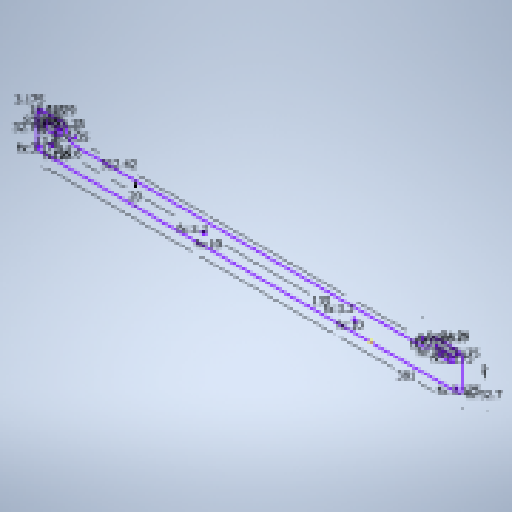
# Autodesk Inventor part: Middle Slide
Saved by Autodesk Inventor 2023 (Build 270158000, 158)
## iProperties
Created: 2022-09-10
Part Number: Middle Slide
Material: Generic
Document SubType Name: Modeling
Designer: deli
Density: 1 g/cm^3
Appearance: Default
Author: deli
Autodesk Inventor part; units mm, degrees
ref_plane "YZ Plane" through (0, 0, 0) normal (1, 0, 0) x (0, 1, 0)
ref_plane "XZ Plane" through (0, 0, 0) normal (0, 1, 0) x (-1, 0, 0)
ref_plane "XY Plane" through (0, 0, 0) normal (0, 0, 1) x (1, 0, 0)
sketch "Sketch1" plane through (0, 0, 0) normal (0, 0, 1) x (1, 0, 0)
  arc A0 (81, 29.525) -> (77.825, 32.7) centre (77.825, 29.525) ccw
  line L0 (77.825, 32.7) -> (59.41, 32.7)
  arc A1 (59.41, 32.7) -> (53.06, 26.35) centre (59.41, 26.35) ccw
  arc A2 (46.71, 20) -> (53.06, 26.35) centre (46.71, 26.35) ccw
  line L1 (46.71, 20) -> (-265.71, 20)
  arc A3 (-272.06, 26.35) -> (-265.71, 20) centre (-265.71, 26.35) ccw
  arc A4 (-272.06, 26.35) -> (-278.41, 32.7) centre (-278.41, 26.35) ccw
  line L2 (-278.41, 32.7) -> (-296.825, 32.7)
  arc A5 (-296.825, 32.7) -> (-300, 29.525) centre (-296.825, 29.525) ccw
  line L3 (-300, 29.525) -> (-300, 3.175)
  arc A6 (-300, 3.175) -> (-296.825, 0) centre (-296.825, 3.175) ccw
  line L4 (-296.825, 0) -> (77.825, 0)
  arc A7 (77.825, 0) -> (81, 3.175) centre (77.825, 3.175) ccw
  line L5 (81, 3.175) -> (81, 29.525)
  arc A8 (62.585, 26.35) -> (62.585, 20) centre (62.585, 23.175) ccw
  line L6 (62.585, 26.35) -> (71.475, 26.35)
  arc A9 (71.475, 20) -> (71.475, 26.35) centre (71.475, 23.175) ccw
  line L7 (71.475, 20) -> (62.585, 20)
  line L8 (-290.475, 26.35) -> (-281.585, 26.35)
  arc A10 (-281.585, 20) -> (-281.585, 26.35) centre (-281.585, 23.175) ccw
  line L9 (-281.585, 20) -> (-290.475, 20)
  arc A11 (-290.475, 26.35) -> (-290.475, 20) centre (-290.475, 23.175) ccw
  circle A12 centre (-151.6, 10) radius 1.6
  circle A13 centre (-286.6, 10) radius 1.6
  circle A14 centre (-16.6, 10) radius 1.6
  point P0 (0, 0)
  point P1 (-272.06, 26.35)
  point P2 (-300, 3.175)
  point P3 (-296.825, 0)
  point P4 (77.825, 0)
  point P5 (62.585, 26.35)
  dimension "d0" = 3.175
  dimension "d1" = 6.35
  dimension "d2" = 3.175
  dimension "d3" = 3.175
  dimension "d4" = 32.7
  dimension "d5" = 34.29
  dimension "d6" = 6.35
  dimension "d7" = 381
  dimension "d8" = 312.42
  dimension "d9" = 34.29
  dimension "d10" = 32.7
  dimension "d11" = 3.175
  dimension "d12" = 3.175
  dimension "d13" = 3.2
  dimension "d14" = 3.2
  dimension "d15" = 3.2
  dimension "d16" = 20
  dimension "d17" = 6.35
  dimension "d18" = 13.4
  dimension "d19" = 10
  dimension "d20" = 10
  dimension "d21" = 10
  dimension "d22" = 6.35
  dimension "d23" = 9.525
  dimension "d24" = 8.89
  dimension "d25" = 3.175
  dimension "d26" = 3.175
  dimension "d27" = 3.175
  dimension "d28" = 6.35
  dimension "d29" = 6.35
  dimension "d30" = 18.415
  dimension "d31" = 18.415
  dimension "d32" = 135
  dimension "d33" = 135
  constraints: 24 point on circle, 20 end point, 15 centre point, 2 tangent, 1 perpendicular
  measures "d0" radius of A5
  measures "d1" radius of A4
  measures "d2" radius of A11
  measures "d3" radius of A10
  measures "d4" distance between parallel lines of L4 L2
  measures "d5" distance from line of L1.end L3
  measures "d6" radius of A3
  measures "d7" distance between parallel lines of L5 L3
  measures "d8" distance of L1.start L1.end
  measures "d9" distance from line of L5 A2.start
  measures "d10" distance between parallel lines of L4 L0
  measures "d11" radius of A8
  measures "d12" radius of A9
  measures "d13" diameter of A13
  measures "d14" diameter of A12
  measures "d15" diameter of A14
  measures "d16" distance between parallel lines of L4 L1
  measures "d17" distance between parallel lines of L8 L9
  measures "d18" distance from line of A13.centre L3
  measures "d19" distance from line of L4 A13.centre
  measures "d20" distance from line of L4 A12.centre
  measures "d21" distance from line of L4 A14.centre
  measures "d22" distance between parallel lines of L2 L8
  measures "d23" distance from line of L3 A11.centre
  measures "d24" distance of L8.start L8.end
  measures "d25" radius of A6
  measures "d26" radius of A7
  measures "d27" radius of A0
  measures "d28" radius of A1
  measures "d29" radius of A2
  measures "d30" distance of L2.start L2.end
  measures "d31" distance of L0.start L0.end
  measures "d32" distance of A13.centre A12.centre
  measures "d33" distance of A14.centre A12.centre
extrude "Extrusion1" add sketch "Sketch1" along normal blind 6.35
sketch "Sketch2" plane through (-296.825, 32.7, 0) normal (0, 1, 0) x (1, 0, 0)
  line L0 (18.415, 0) -> (0, 0) projected
  line L1 (0, 0) -> (0, -6.35) projected
  line L2 (18.415, -6.35) -> (0, -6.35) projected
  line L3 (18.415, 0) -> (18.415, -6.35) projected
  line L4 (374.65, 0) -> (356.235, 0) projected
  line L5 (356.235, 0) -> (356.235, -6.35) projected
  line L6 (374.65, -6.35) -> (356.235, -6.35) projected
  line L7 (374.65, 0) -> (374.65, -6.35) projected
  circle A0 centre (365.4425, -3.175) radius 1.5
  circle A1 centre (9.2075, -3.175) radius 1.5
  point P0 (296.825, 0)
  dimension "d36" = 3
  dimension "d37" = 3
  dimension "d38" = 3.175
  dimension "d39" = 6.35
  dimension "d40" = 18.415
  dimension "d41" = 9.2075
  dimension "d42" = 3.175
  dimension "d43" = 9.2075
  constraints: 2 centre point
  measures "d36" diameter of A0
  measures "d37" diameter of A1
  measures "d38" distance from line of L0 A1.centre
  measures "d39" distance of L0.end L1.end
  measures "d40" distance of L0.start L0.end
  measures "d41" distance from line of L1 A1.centre
  measures "d42" distance from line of L4 A0.centre
  measures "d43" distance from line of L5 A0.centre
extrude "Extrusion2" cut sketch "Sketch2" against normal blind 20 contours A0 | A1
equation "\"d3\" = d2"
equation "\"d6\" = d1"
equation "\"d9\" = d5"
equation "\"d10\" = d4"
equation "\"d11\" = d2"
equation "\"d12\" = d2"
equation "\"d14\" = d13"
equation "\"d15\" = d13"
equation "\"d19\" = 0.5 * d16"
equation "\"d20\" = d19"
equation "\"d21\" = d19"
equation "\"d25\" = d0"
equation "\"d26\" = d0"
equation "\"d27\" = d0"
equation "\"d28\" = d1"
equation "\"d29\" = d1"
equation "\"d31\" = d30"
equation "\"d33\" = d32"
equation "\"d38\" = 0.5 * d39"
equation "\"d41\" = 0.5 * d40"
equation "\"d42\" = d38"
equation "\"d43\" = d41"
body "Solid1"
